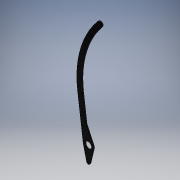
# Autodesk Inventor part: ハンド
Saved by Autodesk Inventor 2019.4 (Build 234330000, 330)
## iProperties
Created: 2021-12-06
Part Number: ハンド
Material: アセタール樹脂、黒
Document SubType Name: Modeling
Designer: 堀川皓史
Density: 1.425 g/cm^3
Appearance: 滑らか - 黒
Mass: 26.787 g
Surface Area: 154.147 cm^2
Volume: 18.7979 cm^3
Author: 堀川皓史
Autodesk Inventor part; units mm, degrees
ref_plane "YZ Plane" through (0, 0, 0) normal (1, 0, 0) x (0, 1, 0)
ref_plane "XZ Plane" through (0, 0, 0) normal (0, 1, 0) x (-1, 0, 0)
ref_plane "XY Plane" through (0, 0, 0) normal (0, 0, 1) x (1, 0, 0)
sketch "スケッチ1" plane through (0, 0, 0) normal (0, 0, 1) x (1, 0, 0)
  circle A0 centre (0, 0) radius 1.6
  circle A1 centre (0, 45) radius 9.55
  line L0 (0, 0) -> (0, 45) construction
  line L1 (0, 45) -> (38.9982, 362.6148) construction
  arc A2 (38.9982, 362.6148) -> (-16.4764, 170.4134) centre (231.3937, 202.9777) ccw
  line L2 (0, 45) -> (-6.5129, 94.574) construction
  arc A3 (-16.4764, 170.4134) -> (6.0935, 94.6273) centre (231.3937, 202.9777) ccw construction
  arc A4 (-14.6969, 42) -> (14.6249, 41.6667) centre (0, 45) ccw construction
  arc A5 (4.875, -1.1111) -> (-4.875, -1.1111) centre (0, 0) ccw construction
  line L3 (-14.7808, 42.3506) -> (-4.875, -1.1111)
  line L4 (14.6249, 41.6667) -> (4.875, -1.1111)
  line L5 (13.601, 51.3255) -> (-6.5129, 94.574)
  line L6 (-6.5129, 94.574) -> (-16.4764, 170.4134)
  arc A6 (38.9982, 362.6148) -> (27.4545, 372.193) centre (33.2263, 367.4039) ccw
  arc A7 (27.4545, 372.193) -> (-31.3486, 168.4596) centre (231.3937, 202.9777) ccw
  line L7 (-31.3486, 168.4596) -> (-14.7808, 42.3506)
  arc A8 (13.601, 51.3255) -> (-14.2261, 40.2443) centre (0, 45) ccw construction
  arc A9 (14.6249, 41.6667) -> (13.601, 51.3255) centre (0, 45) ccw
  arc A10 (-4.875, -1.1111) -> (4.875, -1.1111) centre (0, 0) ccw
  circle A11 centre (33.2263, 367.4039) radius 1.6
  arc A12 (41.0983, 369.7011) -> (-20.1506, 175.8768) centre (231.3937, 202.9777) ccw construction
  arc A13 (32.7138, 373.7709) -> (-17.6145, 121.4982) centre (231.3937, 202.9777) ccw construction
  circle A14 centre (11.9561, 328.899) radius 1.6
  circle A15 centre (-14.4042, 293.6829) radius 1.6
  circle A16 centre (-17.2387, 249.7852) radius 1.6
  circle A17 centre (-30.5608, 207.8618) radius 1.6
  circle A18 centre (-18.8107, 165.471) radius 1.6
  circle A19 centre (11.9561, 328.899) radius 3 construction
  circle A20 centre (-14.4042, 293.6829) radius 3 construction
  circle A21 centre (-17.6145, 121.4982) radius 1.6
  line L8 (-25.0506, 120.5212) -> (-17.6145, 121.4982) construction
  line L9 (-17.6145, 121.4982) -> (-10.1784, 122.4751) construction
  line L10 (33.2263, 367.4039) -> (11.9561, 328.899) construction
  line L11 (11.9561, 328.899) -> (-14.4042, 293.6829) construction
  line L12 (-14.4042, 293.6829) -> (-17.2387, 249.7852) construction
  line L13 (-17.2387, 249.7852) -> (-30.5608, 207.8618) construction
  line L14 (-30.5608, 207.8618) -> (-18.8107, 165.471) construction
  line L15 (-18.8107, 165.471) -> (-17.6145, 121.4982) construction
  dimension "d0" = 3.2
  dimension "d1" = 19.1
  dimension "d2" = 45
  dimension "d3" = 173
  dimension "d4" = 250
  dimension "d6" = 50
  dimension "d7" = 320
  dimension "d8" = 30
  dimension "d9" = 10
  dimension "d10" = 50
  dimension "d11" = 7.5
  dimension "d12" = 3.2
  dimension "d13" = 3.2
  dimension "d14" = 3.2
  dimension "d15" = 3.2
  dimension "d16" = 3.2
  dimension "d17" = 3.2
  dimension "d18" = 6
  dimension "d19" = 6
  dimension "d20" = 3.2
  constraints: 32 end point, 28 point on circle, 22 centre point, 21 tangent, 10 coincident, 6 equal length, 3 point on line, 2 perpendicular, 1 parallel, 1 vertical, 1 vertical alignment
  measures "d0" diameter of A0
  measures "d1" diameter of A1
  measures "d2" distance of point (0, 0) L0.end
  measures "d3" angle of L0 L1
  measures "d4" radius of A2
  measures "d6" distance of L0.end A3.end
  measures "d7" distance of L0.end L1.end
  measures "d8" diameter of A4
  measures "d9" diameter of A5
  measures "d10" distance of L0.end L2.end
  measures "d11" radius of A6
  measures "d12" diameter of A11
  measures "d13" diameter of A14
  measures "d14" diameter of A15
  measures "d15" diameter of A16
  measures "d16" diameter of A17
  measures "d17" diameter of A18
  measures "d18" diameter of A19
  measures "d19" diameter of A20
  measures "d20" diameter of A21
extrude "押し出し1" add sketch "スケッチ1" along normal blind 3
